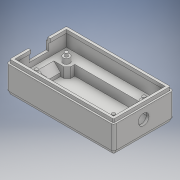
# Autodesk Inventor part: NodeEnclosure
Saved by Autodesk Inventor 2018.3 (Build 223284000, 284)
## iProperties
Created: 2019-03-18
Part Number: NodeEnclosure
Material: Generic
Document SubType Name: Modeling
Designer: matth
Density: 1 g/cm^3
Appearance: Default
Author: matth
Autodesk Inventor part; units mm, degrees
ref_plane "YZ Plane" through (0, 0, 0) normal (1, 0, 0) x (0, 1, 0)
ref_plane "XZ Plane" through (0, 0, 0) normal (0, 1, 0) x (-1, 0, 0)
ref_plane "XY Plane" through (0, 0, 0) normal (0, 0, 1) x (1, 0, 0)
sketch "Sketch1" plane through (0, 0, 0) normal (0, 0, 1) x (1, 0, 0)
  line L0 (-31.3608, 24.9952) -> (32.1392, 24.9952)
  line L1 (32.1392, 24.9952) -> (32.1392, -10.5648)
  line L2 (32.1392, -10.5648) -> (-31.3608, -10.5648)
  line L3 (-31.3608, -10.5648) -> (-31.3608, 24.9952)
  line L4 (30.6392, 23.4952) -> (-29.8608, 23.4952)
  line L5 (-29.8608, 23.4952) -> (-29.8608, -9.0648)
  line L6 (-29.8608, -9.0648) -> (30.6392, -9.0648)
  line L7 (30.6392, -9.0648) -> (30.6392, 23.4952)
  point P0 (0, 0)
  dimension "d0" = 63.5
  dimension "d1" = 35.56
  dimension "d2" = 1.5
  constraints: 16 end point, 4 parallel, 2 perpendicular, 1 horizontal, 3 other
  measures "d0" distance of L1.end L2.end
  measures "d1" distance of L0.end L1.end
  measures "d2" distance between parallel lines of L0 L4
extrude "Extrusion1" add sketch "Sketch1" along normal blind 16.2
sketch "Sketch2" plane through (0, 0, 0) normal (0, 0, -1) x (-1, 0, 0)
  line L0 (-32.1392, -10.5648) -> (31.3608, -10.5648) projected
  line L1 (31.3608, -10.5648) -> (31.3608, 24.9952) projected
  line L2 (31.3608, 24.9952) -> (-32.1392, 24.9952) projected
  line L3 (-32.1392, 24.9952) -> (-32.1392, -10.5648) projected
  point P0 (0, 0)
extrude "Extrusion2" add sketch "Sketch2" along normal blind 1.5
sketch "Sketch3" plane through (0, 0, 0) normal (0, 0, 1) x (1, 0, 0)
  line L0 (-18.6108, 17.2152) -> (19.3892, 17.2152)
  line L1 (19.3892, 17.2152) -> (19.3892, -2.7848)
  line L2 (19.3892, -2.7848) -> (-18.6108, -2.7848)
  line L3 (-18.6108, -2.7848) -> (-18.6108, 17.2152)
  line L4 (30.6392, -9.0648) -> (-29.8608, -9.0648) projected
  line L5 (-29.8608, 23.4952) -> (30.6392, 23.4952) projected
  line L6 (30.6392, 23.4952) -> (30.6392, -9.0648) projected
  line L7 (30.6392, -9.0648) -> (30.6392, 23.4952) projected
  line L8 (30.6392, 23.4952) -> (-29.8608, 23.4952) projected
  line L9 (-29.8608, 23.4952) -> (-29.8608, -9.0648) projected
  line L10 (-29.8608, -9.0648) -> (30.6392, -9.0648) projected
  point P0 (0, 0)
  dimension "d7" = 38
  dimension "d8" = 20
  dimension "d9" = 6.28
  dimension "d10" = 32.56
  dimension "d11" = 11.25
  dimension "d12" = 60.5
  constraints: 8 end point, 2 parallel, 1 horizontal, 1 perpendicular
  measures "d7" distance of L1.end L2.end
  measures "d8" distance of L0.end L1.end
  measures "d9" distance between parallel lines of L4 L2
  measures "d10" distance between parallel lines of L4 L5
  measures "d11" distance between parallel lines of L6 L1
  measures "d12" distance of L4.start L4.end
extrude "Extrusion3" add sketch "Sketch3" along normal blind 6
sketch "Sketch4" plane through (0, 0, 6) normal (0, 0, 1) x (1, 0, 0)
  circle A0 centre (-22.4708, 16.1052) radius 1
  circle A1 centre (-22.4708, -1.6748) radius 1
  circle A2 centre (23.2492, -1.6748) radius 1
  circle A3 centre (23.2489, 16.2887) radius 1
  line L0 (30.6392, -9.0648) -> (-29.8608, -9.0648) projected
  line L1 (-29.8608, 23.4952) -> (30.6392, 23.4952) projected
  line L2 (-29.8608, -9.0648) -> (-29.8608, 23.4952) projected
  point P0 (0, 0)
  dimension "d15" = 2
  dimension "d16" = 2
  dimension "d17" = 2
  dimension "d18" = 2
  dimension "d19" = 45.72
  dimension "d20" = 45.72
  dimension "d21" = 17.78
  dimension "d22" = 7.39
  dimension "d23" = 32.56
  dimension "d24" = 60.5
  dimension "d25" = 7.39
  dimension "d26" = 0
  constraints: 4 centre point
  measures "d15" diameter of A0
  measures "d16" diameter of A1
  measures "d17" diameter of A2
  measures "d18" diameter of A3
  measures "d19" distance of A3.centre A0.centre
  measures "d20" distance of A1.centre A2.centre
  measures "d21" distance of A0.centre A1.centre
  measures "d22" distance from line of L0 A1.centre
  measures "d23" distance between parallel lines of L1 L0
  measures "d24" distance of L0.start L0.end
  measures "d25" distance from line of L2 A1.centre
  measures "d26" horizontal distance of A0.centre A1.centre
extrude "Extrusion4" add sketch "Sketch4" along normal blind 5
sketch "Sketch5" plane through (0, 0, 6) normal (0, 0, 1) x (1, 0, 0)
  circle A0 centre (-22.4708, 16.1052) radius 1 projected
  circle A1 centre (-22.4708, -1.6748) radius 1 projected
  circle A2 centre (23.2492, -1.6748) radius 1 projected
  circle A3 centre (23.2489, 16.2887) radius 1 projected
  circle A4 centre (-22.4708, 16.1052) radius 2
  circle A5 centre (-22.4708, -1.6748) radius 2
  circle A6 centre (23.2492, -1.6748) radius 2
  circle A7 centre (23.2489, 16.2887) radius 2
  point P0 (0, 0)
  dimension "d29" = 1
  dimension "d30" = 1
  dimension "d31" = 1
  dimension "d32" = 1
  constraints: 4 centre point
  measures "d29" radial gap between concentric circles of A0 A4
  measures "d30" radial gap between concentric circles of A1 A5
  measures "d31" radial gap between concentric circles of A2 A6
  measures "d32" radial gap between concentric circles of A3 A7
extrude "Extrusion5" add sketch "Sketch5" along normal blind 3
fillet "Fillet1" radius 1.5 4 edges at (-31.3608, -10.5648, 7.35) (32.1392, -10.5648, 7.35) (32.1392, 24.9952, 7.35) (-31.3608, 24.9952, 7.35)
sketch "Sketch6" plane through (32.1392, -9.0648, 16.2) normal (1, 0, 0) x (0, 0, -1)
  circle A0 centre (8, 16.28) radius 3.2
  line L0 (0, 0) -> (0, 32.56) projected
  line L1 (0, -1.5) -> (17.7, -1.5) projected
  line L2 (17.7, 34.06) -> (0, 34.06) projected
  point P0 (16.2, 9.0648)
  dimension "d36" = 6.4
  dimension "d37" = 8
  dimension "d38" = 17.78
  dimension "d39" = 35.56
  constraints: 1 centre point
  measures "d36" diameter of A0
  measures "d37" distance from line of L0 A0.centre
  measures "d38" distance from line of L1 A0.centre
  measures "d39" distance between parallel lines of L2 L1
extrude "Extrusion6" cut sketch "Sketch6" against normal up to surface (12.75 mm away)
sketch "Sketch7" plane through (19.3892, -2.7848, 0) normal (-1, 0, 0) x (0, 0, 1)
  arc A0 (6, 12.3238) -> (6, 7.6762) centre (8.2, 10) ccw projected
  circle A1 centre (8.2, 10) radius 5.5
  point P0 (0, 2.7848)
  dimension "d42" = 11
  constraints: 1 centre point, 1 coincident
  measures "d42" diameter of A1
extrude "Extrusion7" cut sketch "Sketch7" against normal up to surface (11.25 mm away)
sketch "Sketch8" plane through (0, 0, 6) normal (0, 0, 1) x (1, 0, 0)
  line L0 (-18.6108, -2.7848) -> (-18.6108, 17.2152) projected
  line L1 (-18.6108, 2.4694) -> (-22.595, 2.4694)
  line L2 (-22.595, 2.4694) -> (-22.595, 12.7792)
  line L3 (-22.595, 12.7792) -> (-18.6108, 12.7792)
  line L4 (-18.6108, 12.7792) -> (-18.6108, 2.4694)
  point P0 (0, 0)
  constraints: 8 end point, 2 parallel, 1 horizontal, 1 perpendicular, 1 point on line
extrude "Extrusion8" cut sketch "Sketch8" against normal up to surface (6 mm away)
chamfer "Chamfer1" distance 2 angle 45 2 edges at (-18.6108, 2.4694, 3) (-18.6108, 12.7792, 3)
chamfer "Chamfer2" distance 4 angle 45 1 edges at (-22.595, 7.6243, 6)
sketch "Sketch9" plane through (0, 0, 16.2) normal (0, 0, 1) x (1, 0, 0)
  line L0 (-29.8608, 23.4952) -> (30.6392, 23.4952) projected
  line L1 (-29.8608, -9.0648) -> (-29.8608, 23.4952) projected
  line L2 (30.6392, -9.0648) -> (-29.8608, -9.0648) projected
  line L3 (30.6392, 23.4952) -> (30.6392, -9.0648) projected
  line L4 (29.6392, 22.4952) -> (-28.8608, 22.4952)
  line L5 (-28.8608, 22.4952) -> (-28.8608, -8.0648)
  line L6 (-28.8608, -8.0648) -> (29.6392, -8.0648)
  line L7 (29.6392, -8.0648) -> (29.6392, 22.4952)
  point P0 (0, 0)
  dimension "d53" = 1
  constraints: 8 end point, 3 other
  measures "d53" distance between parallel lines of L0 L4
extrude "Extrusion9" add sketch "Sketch9" against normal blind 3
chamfer "Chamfer3" distance 1 angle 45 4 edges at (-28.8608, 7.2152, 13.2) (0.3892, 22.4952, 13.2) (0.3892, -8.0648, 13.2) (29.6392, 7.2152, 13.2)
sketch "Sketch10" plane through (0, 0, 16.2) normal (0, 0, 1) x (1, 0, 0)
  line L0 (30.6392, 24.9952) -> (-29.8608, 24.9952) projected
  arc A0 (-29.8608, 24.9952) -> (-31.3608, 23.4952) centre (-29.8608, 23.4952) ccw projected
  line L1 (-31.3608, 23.4952) -> (-31.3608, -9.0648) projected
  arc A1 (-31.3608, -9.0648) -> (-29.8608, -10.5648) centre (-29.8608, -9.0648) ccw projected
  line L2 (-29.8608, -10.5648) -> (30.6392, -10.5648) projected
  arc A2 (30.6392, -10.5648) -> (32.1392, -9.0648) centre (30.6392, -9.0648) ccw projected
  line L3 (32.1392, -9.0648) -> (32.1392, 23.4952) projected
  arc A3 (32.1392, 23.4952) -> (30.6392, 24.9952) centre (30.6392, 23.4952) ccw projected
  line L4 (-29.8608, 23.9952) -> (30.6392, 23.9952)
  arc A4 (31.1392, 23.4952) -> (30.6392, 23.9952) centre (30.6392, 23.4952) ccw
  line L5 (31.1392, 23.4952) -> (31.1392, -9.0648)
  arc A5 (30.6392, -9.5648) -> (31.1392, -9.0648) centre (30.6392, -9.0648) ccw
  line L6 (30.6392, -9.5648) -> (-29.8608, -9.5648)
  arc A6 (-30.3608, -9.0648) -> (-29.8608, -9.5648) centre (-29.8608, -9.0648) ccw
  line L7 (-30.3608, -9.0648) -> (-30.3608, 23.4952)
  arc A7 (-29.8608, 23.9952) -> (-30.3608, 23.4952) centre (-29.8608, 23.4952) ccw
  point P0 (0, 0)
  dimension "d59" = 1
  constraints: 8 end point, 8 point on circle, 4 centre point, 7 other
  measures "d59" distance between parallel lines of L0 L4
extrude "Extrusion10" cut sketch "Sketch10" against normal blind 2
sketch "Sketch11" plane through (-31.3608, -9.0648, -1.5) normal (-1, 0, 0) x (0, 0, 1)
  line L0 (17.7, 32.56) -> (17.7, 0) projected
  line L1 (10.7, 22.06) -> (17.7, 22.06)
  line L2 (17.7, 22.06) -> (17.7, 10.5)
  line L3 (17.7, 10.5) -> (10.7, 10.5)
  line L4 (10.7, 10.5) -> (10.7, 22.06)
  line L5 (15.7, 34.06) -> (0, 34.06) projected
  line L6 (0, -1.5) -> (15.7, -1.5) projected
  point P0 (1.5, 9.0648)
  dimension "d62" = 12
  dimension "d63" = 12
  dimension "d64" = 7
  constraints: 8 end point, 2 parallel, 1 horizontal, 1 perpendicular, 1 point on line
  measures "d62" distance between parallel lines of L5 L1
  measures "d63" distance between parallel lines of L6 L3
  measures "d64" distance between parallel lines of L0 L4
extrude "Extrusion11" cut sketch "Sketch11" against normal up to surface (2.5 mm away)
chamfer "Chamfer4" distance 1 distance2 2 8 edges at (0.3892, -10.5648, -1.5) (-30.9214, -10.1255, -1.5) (-31.3608, 7.2152, -1.5) (-30.9214, 24.5559, -1.5) (0.3892, 24.9952, -1.5) (31.6999, 24.5559, -1.5) (32.1392, 7.2152, -1.5) (31.6999, -10.1255, -1.5) measured on face at (-9.6941, 13.1419, -1.5)
equation "\"d9\" = -0.5 * d8 + 0.5 * d10"
equation "\"d11\" = -0.5 * d7 + 0.5 * d12"
equation "\"d20\" = d19"
equation "\"d22\" = -0.5 * d21 + 0.5 * d23"
equation "\"d25\" = -0.5 * d19 + 0.5 * d24"
equation "\"d38\" = 0.5 * d39"
body "Solid1"
